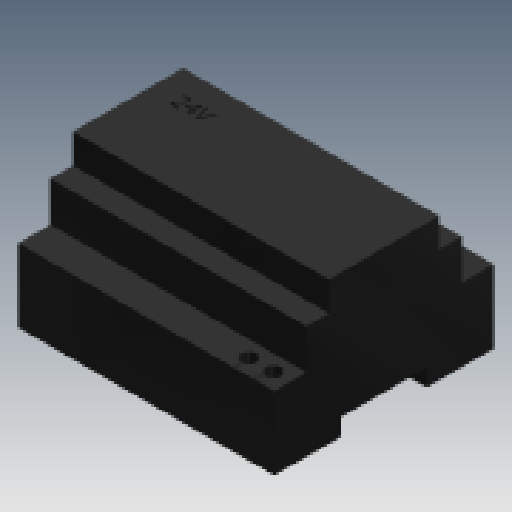
# Autodesk Inventor part: din_pwr_supply
Saved by Autodesk Inventor 2025.4 (Build 294407020, 407B)
## iProperties
Created: 2026-09-08
Part Number: din_pwr_supply
Material: Generic
Document SubType Name: Modeling
Designer: Aiden
Density: 1 g/cm^3
Appearance: Default
Author: Aiden
Autodesk Inventor part; units mm, degrees
ref_plane "YZ Plane" through (0, 0, 0) normal (1, 0, 0) x (0, 1, 0)
ref_plane "XZ Plane" through (0, 0, 0) normal (0, 1, 0) x (-1, 0, 0)
ref_plane "XY Plane" through (0, 0, 0) normal (0, 0, 1) x (1, 0, 0)
sketch "Sketch1" plane through (0, 0, 0) normal (0, 1, 0) x (-1, 0, 0)
  line L0 (0, 0) -> (-105, 0)
  line L1 (-105, 0) -> (-105, -90)
  line L2 (-105, -90) -> (0, -90)
  line L3 (0, -90) -> (0, 0)
  dimension "d0" = 105
  dimension "d1" = 90
  constraints: 8 end point, 2 parallel, 1 horizontal, 1 perpendicular
  measures "d0" distance of L1.end L2.end
  measures "d1" distance of L2.end L0.start
extrude "Extrusion1" add sketch "Sketch1" along normal blind 62.1
sketch "Sketch2" plane through (105, 0, 0) normal (1, 0, 0) x (0, 0, -1)
  line L0 (0, 0) -> (0, 30)
  line L1 (0, 0) -> (0, 62.1) projected
  line L2 (13.175, 30) -> (0, 30)
  line L3 (13.175, 30) -> (13.175, 46.4)
  line L4 (13.175, 46.4) -> (22.425, 46.4)
  line L5 (0, 0) -> (90, 0) projected
  line L6 (90, 0) -> (90, 62.1) projected
  line L7 (0, 62.1) -> (90, 62.1) construction
  line L8 (0, 0) -> (0, 62.1) projected
  line L9 (45, 62.1) -> (45, 0) construction
  line L10 (0, 0) -> (90, 0) projected
  line L11 (45, 0) -> (0, 0)
  line L12 (0, 62.1) -> (90, 62.1) projected
  line L13 (45, 0) -> (0, 0)
  line L14 (22.425, 46.4) -> (22.425, 58.4)
  line L15 (22.425, 58.4) -> (45, 58.4)
  line L16 (90, 0) -> (90, 62.1)
  line L17 (76.825, 30) -> (90, 30)
  line L18 (76.825, 30) -> (76.825, 46.4)
  line L19 (76.825, 46.4) -> (67.575, 46.4)
  line L20 (90, 0) -> (0, 0)
  line L21 (90, 0) -> (0, 0)
  line L22 (45, 0) -> (90, 0)
  line L23 (45, 0) -> (90, 0)
  line L24 (67.575, 46.4) -> (67.575, 58.4)
  line L25 (67.575, 58.4) -> (45, 58.4)
  point P0 (22.425, 52.4)
  point P1 (67.575, 52.4)
  point P2 (90, 30)
  dimension "d4" = 31.825
  dimension "d6" = 22.575
  dimension "d7" = 58.4
  dimension "d8" = 12
  dimension "d9" = 30
  dimension "d10" = 16.4
  constraints: 38 end point, 10 symmetric about line, 3 midpoint, 3 perpendicular, 3 point on line, 2 vertical, 1 collinear, 1 horizontal
  measures "d4" distance between parallel lines of L9 L3
  measures "d6" distance from line of L9 point (22.425, 52.4)
  measures "d7" distance between parallel lines of L11 L15
  measures "d8" distance of L4.end L14.end
  measures "d9" distance of L0.start L0.end
  measures "d10" distance of L2.start L3.end
extrude "Extrusion2" cut sketch "Sketch2" against normal through all contours L1 L12 L6 L17 L18 L19 L24 L25 L15 L14 L4 L3 L2
sketch "Sketch3" plane through (105, 30, 0) normal (0, 1, 0) x (1, 0, 0)
  line L0 (0, 0) -> (0, 90) construction
  line L1 (0, 13.175) -> (0, 0)
  line L2 (-105, 90) -> (-105, 0) projected
  line L3 (-105, 6.5875) -> (0, 6.5875) construction
  circle A0 centre (-7, 6.5875) radius 3.25
  circle A1 centre (-17, 6.5875) radius 3.25
  dimension "d13" = 6.5
  dimension "d14" = 6.5
  dimension "d15" = 7
  dimension "d16" = 10
  constraints: 4 end point, 3 point on line, 2 centre point, 1 midpoint, 1 vertical
  measures "d13" diameter of A0
  measures "d14" diameter of A1
  measures "d15" distance from line of L0 A0.centre
  measures "d16" distance of A0.centre A1.centre
extrude "Extrusion3" cut sketch "Sketch3" against normal blind 10
sketch "Sketch4" plane through (105, 30, -76.825) normal (0, 1, 0) x (1, 0, 0)
  line L0 (-105, 13.175) -> (-105, 0) construction
  line L1 (-105, 6.5875) -> (0, 6.5875) construction
  line L2 (0, -76.825) -> (0, 13.175) projected
  circle A0 centre (-95, 6.5875) radius 2
  circle A1 centre (-91.5, 6.5875) radius 2
  circle A2 centre (-88, 6.5875) radius 2
  circle A3 centre (-84.5, 6.5875) radius 2
  circle A4 centre (-77.5, 6.5875) radius 3.5
  point P0 (-105, -76.825)
  point P1 (-93.25, 7.5557)
  point P2 (-93.25, 5.6193)
  point P3 (-89.75, 5.6193)
  point P4 (-86.25, 5.6193)
  point P5 (-86.25, 7.5557)
  point P6 (-89.75, 7.5557)
  dimension "d19" = 10
  dimension "d20" = 4
  dimension "d23" = 3.5
  dimension "d28" = 7
  dimension "d29" = 7
  constraints: 5 centre point, 4 end point, 3 point on line, 2 horizontal, 1 midpoint, 1 vertical, 6 other
  measures "d19" distance from line of L0 A0.centre
  measures "d20" diameter of A0
  measures "d23" distance of A0.centre A1.centre
  measures "d28" diameter of A4
  measures "d29" distance of A3.centre A4.centre
extrude "Extrusion4" cut sketch "Sketch4" against normal blind 10
sketch "Sketch7" plane through (105, 0, 0) normal (1, 0, 0) x (0, 0, -1)
  line L0 (67.575, 58.4) -> (22.425, 58.4) projected
  line L1 (45, 58.4) -> (45, 0) construction
  line L2 (0, 0) -> (90, 0) projected
  line L3 (27.5, 7) -> (62.5, 7)
  line L4 (62.5, 7) -> (62.5, 0)
  line L5 (62.5, 0) -> (27.5, 0)
  line L6 (27.5, 0) -> (27.5, 7)
  line L7 (27.5, 7) -> (62.5, 0) construction
  line L8 (62.5, 7) -> (27.5, 0) construction
  point P0 (45, 3.5)
  dimension "d36" = 7
  dimension "d37" = 35
  constraints: 14 end point, 4 midpoint, 2 parallel, 2 point on line, 1 horizontal, 1 perpendicular
  measures "d36" distance of L5.end L3.start
  measures "d37" distance of L3.start L3.end
extrude "Extrusion5" cut sketch "Sketch7" against normal through all
sketch "Sketch5" plane through (105, 46.4, -67.575) normal (0, 1, 0) x (1, 0, 0)
  line L0 (-100.4604, 7.4842) -> (-79.0404, 7.4842) construction
  line L1 (-79.0404, 7.4842) -> (-79.0404, 4.7037) construction
  line L2 (-79.0404, 4.7037) -> (-100.4604, 4.7037) construction
  line L3 (-100.4604, 4.7037) -> (-100.4604, 7.4842) construction
  line L4 (-99.1216, 6.101) -> (-100.2751, 6.101)
  line L5 (-100.2751, 6.101) -> (-100.2751, 6.4715)
  line L6 (-100.2751, 6.4715) -> (-99.1216, 6.4715)
  line L7 (-99.1216, 6.4715) -> (-99.1216, 6.101)
  line L8 (-96.864, 7.2397) -> (-97.7261, 4.9525)
  line L9 (-97.7261, 4.9525) -> (-98.0719, 4.9525)
  line L10 (-98.0719, 4.9525) -> (-98.9265, 7.2397)
  line L11 (-98.9265, 7.2397) -> (-98.5091, 7.2397)
  line L12 (-98.5091, 7.2397) -> (-97.8842, 5.4786)
  line L13 (-97.8842, 5.4786) -> (-97.2642, 7.2397)
  line L14 (-97.2642, 7.2397) -> (-96.864, 7.2397)
  line L15 (-94.2038, 6.101) -> (-95.3573, 6.101)
  line L16 (-95.3573, 6.101) -> (-95.3573, 6.4715)
  line L17 (-95.3573, 6.4715) -> (-94.2038, 6.4715)
  line L18 (-94.2038, 6.4715) -> (-94.2038, 6.101)
  line L19 (-91.9462, 7.2397) -> (-92.8083, 4.9525)
  line L20 (-92.8083, 4.9525) -> (-93.1541, 4.9525)
  line L21 (-93.1541, 4.9525) -> (-94.0087, 7.2397)
  line L22 (-94.0087, 7.2397) -> (-93.5913, 7.2397)
  line L23 (-93.5913, 7.2397) -> (-92.9663, 5.4786)
  line L24 (-92.9663, 5.4786) -> (-92.3464, 7.2397)
  line L25 (-92.3464, 7.2397) -> (-91.9462, 7.2397)
  line L26 (-87.8954, 6.1233) -> (-88.9279, 6.1233)
  line L27 (-88.9279, 6.1233) -> (-88.9279, 5.0908)
  line L28 (-88.9279, 5.0908) -> (-89.2687, 5.0908)
  line L29 (-89.2687, 5.0908) -> (-89.2687, 6.1233)
  line L30 (-89.2687, 6.1233) -> (-90.3012, 6.1233)
  line L31 (-90.3012, 6.1233) -> (-90.3012, 6.4518)
  line L32 (-90.3012, 6.4518) -> (-89.2687, 6.4518)
  line L33 (-89.2687, 6.4518) -> (-89.2687, 7.4842)
  line L34 (-89.2687, 7.4842) -> (-88.9279, 7.4842)
  line L35 (-88.9279, 7.4842) -> (-88.9279, 6.4518)
  line L36 (-88.9279, 6.4518) -> (-87.8954, 6.4518)
  line L37 (-87.8954, 6.4518) -> (-87.8954, 6.1233)
  line L38 (-85.4995, 7.2397) -> (-86.3615, 4.9525)
  line L39 (-86.3615, 4.9525) -> (-86.7073, 4.9525)
  line L40 (-86.7073, 4.9525) -> (-87.562, 7.2397)
  line L41 (-87.562, 7.2397) -> (-87.1445, 7.2397)
  line L42 (-87.1445, 7.2397) -> (-86.5196, 5.4786)
  line L43 (-86.5196, 5.4786) -> (-85.8996, 7.2397)
  line L44 (-85.8996, 7.2397) -> (-85.4995, 7.2397)
  line L45 (-81.4487, 6.1233) -> (-82.4811, 6.1233)
  line L46 (-82.4811, 6.1233) -> (-82.4811, 5.0908)
  line L47 (-82.4811, 5.0908) -> (-82.822, 5.0908)
  line L48 (-82.822, 5.0908) -> (-82.822, 6.1233)
  line L49 (-82.822, 6.1233) -> (-83.8545, 6.1233)
  line L50 (-83.8545, 6.1233) -> (-83.8545, 6.4518)
  line L51 (-83.8545, 6.4518) -> (-82.822, 6.4518)
  line L52 (-82.822, 6.4518) -> (-82.822, 7.4842)
  line L53 (-82.822, 7.4842) -> (-82.4811, 7.4842)
  line L54 (-82.4811, 7.4842) -> (-82.4811, 6.4518)
  line L55 (-82.4811, 6.4518) -> (-81.4487, 6.4518)
  line L56 (-81.4487, 6.4518) -> (-81.4487, 6.1233)
  line L57 (-79.0527, 7.2397) -> (-79.9148, 4.9525)
  line L58 (-79.9148, 4.9525) -> (-80.2606, 4.9525)
  line L59 (-80.2606, 4.9525) -> (-81.1152, 7.2397)
  line L60 (-81.1152, 7.2397) -> (-80.6978, 7.2397)
  line L61 (-80.6978, 7.2397) -> (-80.0729, 5.4786)
  line L62 (-80.0729, 5.4786) -> (-79.4529, 7.2397)
  line L63 (-79.4529, 7.2397) -> (-79.0527, 7.2397)
  point P0 (-105, -67.575)
  constraints: 2 other
emboss "Emboss1" sketch "Sketch5" operation cut depth 2 direction (0, -1, 0)
sketch "Sketch6" plane through (105, 30, 0) normal (0, 1, 0) x (1, 0, 0)
  line L0 (-17.3791, 3.0471) -> (-7.0215, 3.0471) construction
  line L1 (-7.0215, 3.0471) -> (-7.0215, 0.4536) construction
  line L2 (-7.0215, 0.4536) -> (-17.3791, 0.4536) construction
  line L3 (-17.3791, 0.4536) -> (-17.3791, 3.0471) construction
  line L4 (-15.755, 0.4536) -> (-16.9941, 0.4536)
  line L5 (-16.9941, 0.4536) -> (-16.9941, 0.713)
  line L6 (-16.9941, 0.713) -> (-16.5331, 0.713)
  line L7 (-16.5331, 0.713) -> (-16.5331, 2.4152)
  line L8 (-16.5331, 2.4152) -> (-16.9941, 2.4152)
  line L9 (-16.9941, 2.4152) -> (-16.9941, 2.6478)
  spline S0 degree 2 poles (-16.9941, 2.6478) (-16.7327, 2.6478) (-16.4857, 2.796) (-16.4693, 3.0019) knots 0 0 0 1 2 2 2
  line L10 (-16.4693, 3.0019) -> (-16.2058, 3.0019)
  line L11 (-16.2058, 3.0019) -> (-16.2058, 0.713)
  line L12 (-16.2058, 0.713) -> (-15.755, 0.713)
  line L13 (-15.755, 0.713) -> (-15.755, 0.4536)
  line L14 (-7.1758, 0.4536) -> (-8.7422, 0.4536)
  line L15 (-8.7422, 0.4536) -> (-8.7422, 0.8138)
  spline S1 degree 2 poles (-8.7422, 0.8138) (-8.5735, 0.9723) (-8.2729, 1.2667) (-8.1288, 1.4252) knots 0 0 0 1 2 2 2
  spline S2 degree 2 poles (-8.1288, 1.4252) (-7.8386, 1.7442) (-7.6266, 2.1271) (-7.6266, 2.3308) knots 0 0 0 1 2 2 2
  spline S3 degree 2 poles (-7.6266, 2.3308) (-7.6266, 2.4379) (-7.6925, 2.5984) (-7.7522, 2.6499) knots 0 0 0 1 2 2 2
  spline S4 degree 2 poles (-7.7522, 2.6499) (-7.8119, 2.7013) (-7.9683, 2.7528) (-8.063, 2.7528) knots 0 0 0 1 2 2 2
  spline S5 degree 2 poles (-8.063, 2.7528) (-8.1535, 2.7528) (-8.3388, 2.7075) (-8.4232, 2.6725) knots 0 0 0 1 2 2 2
  spline S6 degree 2 poles (-8.4232, 2.6725) (-8.4952, 2.6437) (-8.629, 2.5614) (-8.6702, 2.5326) knots 0 0 0 1 2 2 2
  line L16 (-8.6702, 2.5326) -> (-8.6887, 2.5326)
  line L17 (-8.6887, 2.5326) -> (-8.6887, 2.8948)
  spline S7 degree 2 poles (-8.6887, 2.8948) (-8.5837, 2.9463) (-8.2071, 3.0471) (-8.0383, 3.0471) knots 0 0 0 1 2 2 2
  spline S8 degree 2 poles (-8.0383, 3.0471) (-7.6822, 3.0471) (-7.2808, 2.6705) (-7.2808, 2.3494) knots 0 0 0 1 2 2 2
  spline S9 degree 2 poles (-7.2808, 2.3494) (-7.2808, 2.1991) (-7.3508, 1.948) (-7.4125, 1.841) knots 0 0 0 1 2 2 2
  spline S10 degree 2 poles (-7.4125, 1.841) (-7.4743, 1.7298) (-7.6534, 1.5116) (-7.7522, 1.4066) knots 0 0 0 1 2 2 2
  spline S11 degree 2 poles (-7.7522, 1.4066) (-7.9127, 1.2317) (-8.3059, 0.8571) (-8.4232, 0.748) knots 0 0 0 1 2 2 2
  line L18 (-8.4232, 0.748) -> (-7.1758, 0.748)
  line L19 (-7.1758, 0.748) -> (-7.1758, 0.4536)
  point P0 (-105, 0)
  constraints: 2 other
emboss "Emboss2" sketch "Sketch6" operation cut depth 2 direction (0, -1, 0)
sketch "Sketch8" plane through (105, 58.4, -22.425) normal (0, 1, 0) x (1, 0, 0)
  line L0 (-95.7206, 35.8955) -> (-81.4983, 35.8955) construction
  line L1 (-81.4983, 35.8955) -> (-81.4983, 29.6711) construction
  line L2 (-81.4983, 29.6711) -> (-95.7206, 29.6711) construction
  line L3 (-95.7206, 29.6711) -> (-95.7206, 35.8955) construction
  line L4 (-91.5167, 29.6711) -> (-95.276, 29.6711)
  line L5 (-95.276, 29.6711) -> (-95.276, 30.5356)
  spline S0 degree 2 poles (-95.276, 30.5356) (-94.8709, 30.916) (-94.1497, 31.6224) (-93.8039, 32.0028) knots 0 0 0 1 2 2 2
  spline S1 degree 2 poles (-93.8039, 32.0028) (-93.1073, 32.7685) (-92.5985, 33.6873) (-92.5985, 34.1764) knots 0 0 0 1 2 2 2
  spline S2 degree 2 poles (-92.5985, 34.1764) (-92.5985, 34.4333) (-92.7566, 34.8186) (-92.8999, 34.9421) knots 0 0 0 1 2 2 2
  spline S3 degree 2 poles (-92.8999, 34.9421) (-93.0431, 35.0656) (-93.4186, 35.1891) (-93.6458, 35.1891) knots 0 0 0 1 2 2 2
  spline S4 degree 2 poles (-93.6458, 35.1891) (-93.8632, 35.1891) (-94.3078, 35.0804) (-94.5103, 34.9964) knots 0 0 0 1 2 2 2
  spline S5 degree 2 poles (-94.5103, 34.9964) (-94.6832, 34.9273) (-95.0043, 34.7297) (-95.1031, 34.6605) knots 0 0 0 1 2 2 2
  line L6 (-95.1031, 34.6605) -> (-95.1476, 34.6605)
  line L7 (-95.1476, 34.6605) -> (-95.1476, 35.5299)
  spline S6 degree 2 poles (-95.1476, 35.5299) (-94.8956, 35.6534) (-93.9916, 35.8955) (-93.5865, 35.8955) knots 0 0 0 1 2 2 2
  spline S7 degree 2 poles (-93.5865, 35.8955) (-92.7319, 35.8955) (-91.7686, 34.9915) (-91.7686, 34.2208) knots 0 0 0 1 2 2 2
  spline S8 degree 2 poles (-91.7686, 34.2208) (-91.7686, 33.8602) (-91.9366, 33.2575) (-92.0848, 33.0006) knots 0 0 0 1 2 2 2
  spline S9 degree 2 poles (-92.0848, 33.0006) (-92.233, 32.7339) (-92.6627, 32.2102) (-92.8999, 31.9583) knots 0 0 0 1 2 2 2
  spline S10 degree 2 poles (-92.8999, 31.9583) (-93.2852, 31.5384) (-94.2287, 30.6393) (-94.5103, 30.3775) knots 0 0 0 1 2 2 2
  line L8 (-94.5103, 30.3775) -> (-91.5167, 30.3775)
  line L9 (-91.5167, 30.3775) -> (-91.5167, 29.6711)
  line L10 (-86.7792, 31.7656) -> (-87.5053, 31.7656)
  line L11 (-87.5053, 31.7656) -> (-87.5053, 29.6711)
  line L12 (-87.5053, 29.6711) -> (-88.2908, 29.6711)
  line L13 (-88.2908, 29.6711) -> (-88.2908, 31.7656)
  line L14 (-88.2908, 31.7656) -> (-90.9831, 31.7656)
  line L15 (-90.9831, 31.7656) -> (-90.9831, 32.6252)
  line L16 (-90.9831, 32.6252) -> (-88.2562, 35.7671)
  line L17 (-88.2562, 35.7671) -> (-87.5053, 35.7671)
  line L18 (-87.5053, 35.7671) -> (-87.5053, 32.4227)
  line L19 (-87.5053, 32.4227) -> (-86.7792, 32.4227)
  line L20 (-86.7792, 32.4227) -> (-86.7792, 31.7656)
  line L21 (-88.2908, 32.4227) -> (-88.2908, 34.8038)
  line L22 (-88.2908, 34.8038) -> (-90.3409, 32.4227)
  line L23 (-90.3409, 32.4227) -> (-88.2908, 32.4227)
  line L24 (-81.5328, 35.7671) -> (-83.6324, 29.6711)
  line L25 (-83.6324, 29.6711) -> (-84.5067, 29.6711)
  line L26 (-84.5067, 29.6711) -> (-86.6063, 35.7671)
  line L27 (-86.6063, 35.7671) -> (-85.7368, 35.7671)
  line L28 (-85.7368, 35.7671) -> (-84.0473, 30.7035)
  line L29 (-84.0473, 30.7035) -> (-82.3578, 35.7671)
  line L30 (-82.3578, 35.7671) -> (-81.5328, 35.7671)
  point P0 (-105, -22.425)
  constraints: 2 other
emboss "Emboss3" sketch "Sketch8" operation cut depth 2 direction (0, -1, 0)
equation "\"d17\" = d16"
equation "\"d30\" = d16"
body "Solid1"
